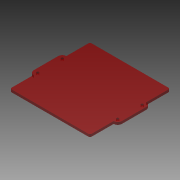
# Autodesk Inventor part: plastic_part_11
Saved by Autodesk Inventor 2013 (Build 170138000, 138)
## iProperties
Shininess: 20.0
Created: 2013-05-22
Part Number: plastic_part_11
Document SubType Name: Modeling
Designer: Noa Izumi
Material: Default
Density: 1 g/cm^3
Density: 0.0
Volumn: 0.0
Area: 0.0
PropertySet Name: Model Information
Control State: 0
Master: False
Checked Out: False
Author: Noa Izumi
Autodesk Inventor part; units mm, degrees
ref_plane "YZ Plane" through (0, 0, 0) normal (1, 0, 0) x (0, 1, 0)
ref_plane "XZ Plane" through (0, 0, 0) normal (0, 1, 0) x (-1, 0, 0)
ref_plane "XY Plane" through (0, 0, 0) normal (0, 0, 1) x (1, 0, 0)
sketch "Sketch1" plane through (0, 0, 0) normal (0, 0, 1) x (1, 0, 0)
  line L0 (0, 0) -> (98, 0)
  line L1 (98, 0) -> (98, 98)
  line L2 (98, 98) -> (0, 98)
  line L3 (0, 98) -> (0, 0)
  line L4 (-5, 69) -> (103, 69)
  line L5 (103, 69) -> (103, 29)
  line L6 (103, 29) -> (-5, 29)
  line L7 (-5, 29) -> (-5, 69)
  dimension "d0" = 98
  dimension "d1" = 98
  dimension "d14" = 108
  dimension "d15" = 40
  dimension "d16" = 5
  dimension "d17" = 29
  constraints: 16 end point, 4 parallel, 2 horizontal, 2 perpendicular
  measures "d0" distance of L0.start L0.end
  measures "d1" distance of L2.end L0.start
  measures "d14" distance of L5.end L6.end
  measures "d15" distance of L6.end L4.start
  measures "d16" distance between parallel lines of L3 L7
  measures "d17" distance between parallel lines of L2 L4
extrude "Extrusion1" add sketch "Sketch1" along normal blind 3
fillet "Fillet3" radius 2 4 edges at (0, 0, 1.5) (98, 0, 1.5) (0, 98, 1.5) (98, 98, 1.5)
fillet "Fillet9" radius 5 4 edges at (-5, 29, 1.5) (-5, 69, 1.5) (103, 29, 1.5) (103, 69, 1.5)
sketch "Sketch8" plane through (0, 0, 3) normal (0, 0, 1) x (1, 0, 0)
  arc A0 (0, 69) -> (-5, 64) centre (0, 64) ccw projected
  arc A1 (-5, 34) -> (0, 29) centre (0, 34) ccw projected
  arc A2 (98, 29) -> (103, 34) centre (98, 34) ccw projected
  arc A3 (103, 64) -> (98, 69) centre (98, 64) ccw projected
  constraints: 4 coincident
hole "Hole5" at (0, 34, 3) at (0, 64, 3) at (98, 34, 3) at (98, 64, 3) direction (0, 0, -1) diameter 3 end through all
